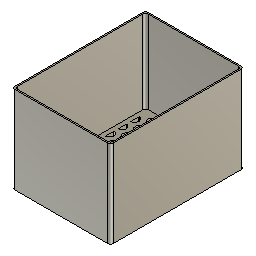
Cheese Box (Autodesk Fusion 360 design; units mm, degrees)
Autodesk Fusion 360 part; units mm, degrees
note: some values were not read from the file. Chosen so that the rebuilt part matches the saved one: which bodies a step acts on; which face or edge a step refers to.
box "BoxPrimitive1" add length 95 width 70 height 60 placed x (0, 1, 0) y (-1, 0, 0) z (0, 0, 1) at (70, 0, 0) makes body 1
shell "Shell1" thickness 1 removed faces 1 at (23.3333, 31.6667, 60) on bodies 1
fillet "Fillet1" radius 2 8 edges at (1, 94, 30.5) (69, 1, 30.5) (69, 94, 30.5) (1, 1, 30.5) (70, 95, 30) (0, 95, 30) (70, 0, 30) (0, 0, 30) on bodies 1
sketch "Sketch3" plane through (0, 0, 0) normal (0, 0, -1) x (1, 0, 0)
  arc A0 (2, 0) -> (0, -2) centre (2, -2) ccw
  line L0 (0, -2) -> (0, -93)
  arc A1 (0, -93) -> (2, -95) centre (2, -93) ccw
  line L1 (2, -95) -> (68, -95)
  arc A2 (68, -95) -> (70, -93) centre (68, -93) ccw
  line L2 (70, -93) -> (70, -2)
  arc A3 (70, -2) -> (68, 0) centre (68, -2) ccw
  line L3 (68, 0) -> (2, 0)
  arc A4 (3, -1) -> (1, -3) centre (3, -3) ccw
  line L4 (3, -1) -> (67, -1)
  arc A5 (69, -3) -> (67, -1) centre (67, -3) ccw
  line L5 (69, -3) -> (69, -92)
  arc A6 (67, -94) -> (69, -92) centre (67, -92) ccw
  line L6 (67, -94) -> (3, -94)
  arc A7 (1, -92) -> (3, -94) centre (3, -92) ccw
  line L7 (1, -92) -> (1, -3)
  line L8 (66, -9) -> (66, -86)
  line L9 (9, -4) -> (61, -4)
  line L10 (4, -86) -> (4, -9)
  line L11 (61, -91) -> (9, -91)
  arc A8 (9, -4) -> (4, -9) centre (9, -9) ccw
  arc A9 (4, -86) -> (9, -91) centre (9, -86) ccw
  arc A10 (66, -9) -> (61, -4) centre (61, -9) ccw
  arc A11 (61, -91) -> (66, -86) centre (61, -86) ccw
  line L12 (35, -4) -> (35, -91) construction
  circle A12 centre (35, -47.5) radius 3
  line L13 (35, -47.5) -> (58.3298, -60.9695)
  dimension "d12" = 5
  dimension "d13" = 6
  dimension "d16" = 60
  constraint tangent L9 A8
  constraint tangent L10 A8
  constraint tangent L11 A9
  constraint tangent L10 A9
  constraint equal A8 A9
  constraint tangent L9 A10
  constraint tangent L8 A10
  constraint equal A8 A10
  constraint tangent L8 A11
  constraint tangent L11 A11
  constraint equal A8 A11
  constraint midpoint L9 L12.start
  constraint midpoint L11 L12.end
  constraint midpoint L12 A12.centre
  constraint coincident A12.centre L13.start
  measures "d12" radius of A8
  measures "d13" diameter of A12
  measures "d16" angle of L12 L13
split "Split1" by curves path "Sketch3" along A11 L11 A9 L10 A8 L9 A10 L8 bodies 1 makes body 2 at (70, 32.3333, 20)
extrude "Extrude1" cut sketch "Sketch3" against normal blind 1 contours A12 bodies 1
pattern_linear "R-Pattern1" count 9 spacing 9 along (0.866025, 0.5, 0) both ways count 13 spacing 9 along (0, 1, 0) both ways of "Extrude1"
combine "Combine1" operation add target body 2 tool bodies 1
move_face "OffsetFaces1" offset 2 1 faces at (4.9796, 90.265, 0) on bodies 2
